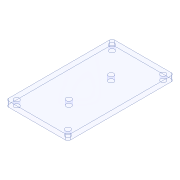
# Autodesk Inventor part: Top&Bottom
Saved by Autodesk Inventor 2020 (Build 240168000, 168)
## iProperties
Created: 2022-03-07
Part Number: Top&Bottom
Material: Generic
Document SubType Name: Modeling
Designer: ferrerx
Density: 1 g/cm^3
Appearance: Clear - Blue
Author: ferrerx
Autodesk Inventor part; units mm, degrees
ref_plane "YZ Plane" through (0, 0, 0) normal (1, 0, 0) x (0, 1, 0)
ref_plane "XZ Plane" through (0, 0, 0) normal (0, 1, 0) x (-1, 0, 0)
ref_plane "XY Plane" through (0, 0, 0) normal (0, 0, 1) x (1, 0, 0)
sketch "Sketch1" plane through (0, 0, 0) normal (0, 1, 0) x (-1, 0, 0)
  line L0 (11.5, 24) -> (-11.5, 24)
  line L1 (-11.5, 24) -> (-11.5, -24)
  line L2 (-11.5, -24) -> (11.5, -24)
  line L3 (11.5, -24) -> (11.5, 24)
  line L4 (11.5, 24) -> (-11.5, -24) construction
  line L5 (-11.5, 24) -> (11.5, -24) construction
  line L6 (-8.5, 21) -> (8.5, 21)
  line L7 (8.5, 21) -> (8.5, -21)
  line L8 (8.5, -21) -> (-8.5, -21)
  line L9 (-8.5, -21) -> (-8.5, 21)
  line L10 (-8.5, 21) -> (8.5, -21) construction
  line L11 (8.5, 21) -> (-8.5, -21) construction
  line L12 (0, 0) -> (-8.5, 0) construction
  circle A0 centre (0, -12) radius 1.5
  circle A1 centre (0, 12) radius 1.5
  line L13 (17.5, 30) -> (-17.5, 30)
  line L14 (-17.5, 30) -> (-17.5, -30)
  line L15 (-17.5, -30) -> (17.5, -30)
  line L16 (17.5, -30) -> (17.5, 30)
  line L17 (17.5, 30) -> (-17.5, -30) construction
  line L18 (-17.5, 30) -> (17.5, -30) construction
  circle A2 centre (14.5, 27) radius 1.5
  circle A3 centre (-14.5, 27) radius 1.5
  circle A4 centre (14.5, -27) radius 1.5
  circle A5 centre (-14.5, -27) radius 1.5
  dimension "d0" = 23
  dimension "d1" = 48
  dimension "d3" = 3
  dimension "d4" = 3
  dimension "d5" = 3
  dimension "d6" = 12
  dimension "d9" = 6
  dimension "d10" = 6
  dimension "d13" = 3
  dimension "d14" = 3
  dimension "d15" = 3
  dimension "d16" = 3
  dimension "d17" = 3
  dimension "d18" = 3
  constraints: 38 end point, 7 midpoint, 6 centre point, 6 parallel, 3 horizontal, 3 perpendicular, 3 symmetric about line, 3 other
  measures "d0" distance of L1.end L2.end
  measures "d1" distance of L0.end L1.end
  measures "d3" distance between parallel lines of L2 L8
  measures "d4" distance between parallel lines of L3 L7
  measures "d5" diameter of A0
  measures "d6" distance from line of L12 A0.centre
  measures "d9" distance between parallel lines of L1 L14
  measures "d10" distance between parallel lines of L2 L15
  measures "d13" diameter of A2
  measures "d14" distance from line of L13 A2.centre
  measures "d15" distance from line of L16 A2.centre
  measures "d16" diameter of A3
  measures "d17" distance from line of L13 A3.centre
  measures "d18" distance from line of L14 A3.centre
extrude "Extrusion1" add sketch "Sketch1" along normal blind 3 contours L3 L2 L1 L0 | L6 L7 L8 L9 | L16 L15 L14 L13
fillet "Fillet2" radius 1.5 4 edges at (17.5, 1.5, -30) (17.5, 1.5, 30) (-17.5, 1.5, 30) (-17.5, 1.5, -30)
body "Solid1"
